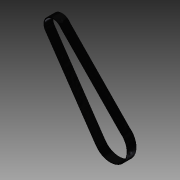
# Autodesk Inventor part: z-belt
Saved by Autodesk Inventor 2013 SP2 (Build 170200200, 200)
## iProperties
Created: 2013-02-27
Part Number: z-belt
Material: Generic
Document SubType Name: Modeling
Designer: Edward
Density: 1 g/cm^3
Description: 188mm GT2, 6mm wide continuous belting
Mass: 0.745461 g
Surface Area: 26.3625 cm^2
Volume: 0.745461 cm^3
Vendor: custom
Author: Edward
Autodesk Inventor part; units mm, degrees
ref_plane "YZ Plane" through (0, 0, 0) normal (1, 0, 0) x (0, 1, 0)
ref_plane "XZ Plane" through (0, 0, 0) normal (0, 1, 0) x (-1, 0, 0)
ref_plane "XY Plane" through (0, 0, 0) normal (0, 0, 1) x (1, 0, 0)
sketch "Sketch1" plane through (0, 0, 0) normal (0, 0, 1) x (1, 0, 0)
  arc A0 (-6.3312, 9.4953) -> (-1.2535, 11.3435) centre (0, 0) ccw projected
  arc A1 (-39.762, 56.0914) -> (-36.7433, 54.5415) centre (-40.9824, 50) ccw projected
  arc A2 (-35.5994, 53.3683) -> (-45.7281, 45.7808) centre (-40.9824, 50) ccw
  arc A3 (-9.826, -6.7195) -> (7.1791, 9.4953) centre (0, 0) ccw
  line L0 (-45.7281, 45.7808) -> (-9.826, -6.7195)
  line L1 (-36.7433, 54.5415) -> (-36.3354, 54.1231)
  line L2 (-35.5994, 53.3683) -> (7.1791, 9.4953)
  arc A4 (-10.3384, -7.0699) -> (7.5913, 9.9618) centre (0, 0) ccw
  line L3 (-10.3384, -7.0699) -> (-46.2188, 45.3986)
  arc A5 (-35.1095, 53.7552) -> (-46.2188, 45.3986) centre (-40.9824, 50) ccw
  line L4 (-35.1095, 53.7552) -> (7.5913, 9.9618)
  point P0 (0, 0)
  dimension "d0" = 12.7
  constraints: 10 end point, 9 point on circle, 4 centre point, 2 coincident, 1 tangent, 3 other
  measures "d0" diameter of A2
extrude "Extrusion1" add sketch "Sketch1" along normal blind 6.35 contours L3 A5 L4 A4
body "Solid1"
